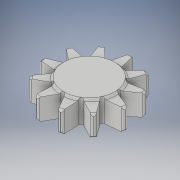
# Autodesk Inventor part: engrenage_roation_1
Saved by Autodesk Inventor 2019 (Build 230136000, 136)
## iProperties
Created: 2018-05-18
Part Number: engrenage_roation_1
Material: Générique
Document SubType Name: Modeling
Designer: Theo
Density: 1 g/cm^3
Appearance: Par défaut
Author: Theo
Autodesk Inventor part; units mm, degrees
ref_plane "YZ Plane" through (0, 0, 0) normal (1, 0, 0) x (0, 1, 0)
ref_plane "XZ Plane" through (0, 0, 0) normal (0, 1, 0) x (-1, 0, 0)
ref_plane "XY Plane" through (0, 0, 0) normal (0, 0, 1) x (1, 0, 0)
sketch "Esquisse1" plane through (0, 0, 0) normal (1, 0, 0) x (0, 1, 0)
  line L0 (-20.5129, 0) -> (20.5129, 0)
  line L1 (4.5, 10) -> (5, 9.5)
  line L2 (5, 9.5) -> (5, 6.5)
  line L3 (4.5, 10) -> (0.5, 10)
  line L4 (0.5, 10) -> (0, 9.5)
  line L5 (0, 9.5) -> (0, 0)
  line L6 (0, 0) -> (5.5, 0)
  line L7 (5.5, 0) -> (5.5, 6)
  line L8 (5.5, 6) -> (5, 6.5)
  dimension "d0" = 5
  dimension "d1" = 0.5
  dimension "d2" = 0.5
  dimension "d3" = 0.5
  dimension "d4" = 0.5
  dimension "d5" = 20
  dimension "d17" = 0.5
  dimension "d18" = 0.5
  dimension "d19" = 12
  constraints: 18 end point, 3 horizontal, 3 vertical, 1 coincident, 1 midpoint
  measures "d0" distance between parallel lines of L2 L5
  measures "d1" horizontal distance of L1.start L1.end
  measures "d2" horizontal distance of L1.start L1.end
  measures "d3" horizontal distance of L3.end L4.end
  measures "d4" horizontal distance of L3.end L4.end
  measures "d5" diameter of L3 L0
  measures "d17" horizontal distance of L2.end L7.end
  measures "d18" horizontal distance of L2.end L7.end
  measures "d19" diameter of L7.end L0
revolve "Révolution1" add sketch "Esquisse1" angle 360 about axis through (0, -20.5129, 0) along (0, 1, 0)
sketch "Esquisse2" plane through (0, 5.5, 0) normal (0, 1, 0) x (1, 0, 0)
  circle A0 centre (0, 0) radius 10 construction
  arc A1 (0.433, -6.25) -> (-0.433, -6.25) centre (0, -6.5) ccw
  line L0 (0.433, -6.25) -> (2.2333, -9.3682)
  line L1 (-0.433, -6.25) -> (-2.2333, -9.3682)
  arc A2 (-2.8066, -9.5981) -> (-2.2333, -9.3682) centre (-2.6663, -9.1182) ccw
  arc A3 (2.2333, -9.3682) -> (2.8066, -9.5981) centre (2.6663, -9.1182) ccw
  arc A4 (-2.8066, -9.5981) -> (2.8066, -9.5981) centre (0, 0) ccw
  point P0 (0, 0)
  point P1 (0, -10)
  dimension "d8" = 60
  dimension "d9" = 0.5
  dimension "d10" = 0.5
  dimension "d11" = 3.5
  constraints: 11 point on circle, 6 tangent, 4 centre point, 4 end point, 2 vertical alignment, 1 coincident, 1 equal length, 1 equal radius
  measures "d8" angle of L0 L1
  measures "d9" radius of A2
  measures "d10" radius of A1
  measures "d11" distance of A1.centre A0.start
extrude "Extrusion1" cut sketch "Esquisse2" against normal up to surface (5.5 mm away)
pattern_circular "Réseau circulaire1" count 11 over 360 about axis through (0, -10, 0) along (0, 1, 0) of "Extrusion1"
equation "\"d2\" = d1"
equation "\"d3\" = d1"
equation "\"d4\" = d1"
